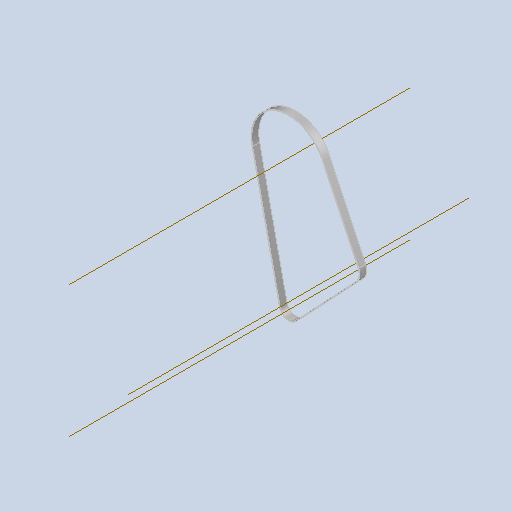
# Autodesk Inventor part: Synchronous Belt
Saved by Autodesk Inventor 2024 (Build 280153000, 153)
## iProperties
Created: 2024-01-05
Part Number: Synchronous Belt
Material: Rubber
Document SubType Name: Modeling
Designer: MaartenGeorgesBuelen
Density: 1 g/cm^3
Appearance: Rubber - Black - Version 1.1
CustomPartVersion: 1
Author: MaartenGeorgesBuelen
Autodesk Inventor part; units mm, degrees
sketch "Sketch Path" plane through (0, 0, 0) normal (0, 0, 1) x (1, 0, 0)
  arc A0 (-7.7726, -1.7064) -> (5.7825, -5.4671) centre (0, 0) ccw
  arc A1 (28.5211, 126.0836) -> (-31.3392, 105.6375) centre (-0.2486, 112.4632) ccw
  arc A2 (57.7606, 49.5098) -> (59.523, 60.6) centre (50.5325, 56.3436) ccw
  line L0 (57.7606, 49.5098) -> (5.7825, -5.4671)
  line L1 (-7.7726, -1.7064) -> (-31.3392, 105.6375)
  line L2 (28.5211, 126.0836) -> (59.523, 60.6)
  constraints: 6 end point, 6 point on circle, 3 centre point
ref_plane "Cross Section Plane" through (5.7825, -5.4671, 0) normal (0.687, 0.7266, 0) x (0, 0, 1)
ref_plane "Work Plane2" through (0, 0, 0) normal (-1, 0, 0) x (0, 0, 1)
ref_plane "Work Plane3" through (-0.2486, 112.4632, 0) normal (0.1583, -0.9874, 0) x (0, 0, 1)
ref_plane "Work Plane4" through (50.5325, 56.3436, 0) normal (-0.2812, 0.9597, 0) x (0, 0, 1)
sketch "Cross Section" plane through (5.7825, -5.4671, 0) normal (0.687, 0.7266, 0) x (0, 0, 1)
  line L0 (-3, 0.3) -> (3, 0.3)
  line L1 (3, 0.3) -> (3, -0.3)
  line L2 (3, -0.3) -> (-3, -0.3)
  line L3 (-3, -0.3) -> (-3, 0.3)
  line L4 (-3, 0) -> (3, 0) construction
  point P0 (0, 0)
  point P1 (0, 0)
  dimension "d0" = 6
  dimension "d4" = 0.3
  dimension "d5" = 0.3
  constraints: 10 end point, 3 midpoint, 2 parallel, 1 coincident, 1 horizontal, 1 perpendicular, 1 other
  measures "d0" distance between parallel lines of L1 L3
  measures "d4" distance between parallel lines of L2 L4
  measures "d5" distance between parallel lines of L4 L0
sweep "Belt" add profiles "Cross Section" path "Sketch Path"
equation "\"d0\" = da_B"
equation "\"d4\" = da_a"
equation "\"d5\" = da_a2"
equation "\"da_B\" = 6"
equation "\"da_pb\" = 2.5"
equation "\"da_a\" = 0.3"
equation "\"da_S\" = 1.5"
equation "\"da_Beta\" = 20deg"
equation "\"da_Ht\" = 0.7"
equation "\"da_H\" = 1.3"
equation "\"da_a2\" = 0.3"
body "Solid1"
